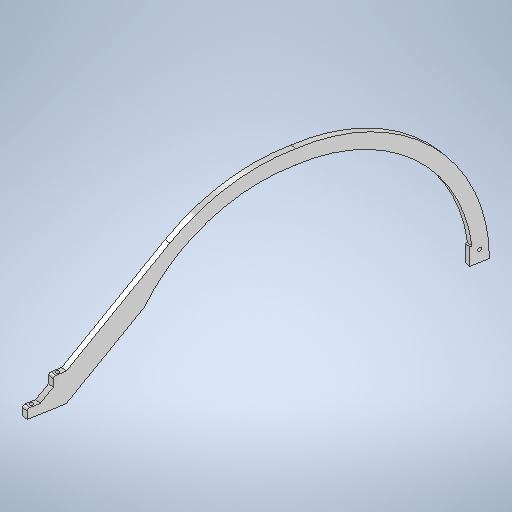
# Autodesk Inventor part: hand2_06
Saved by Autodesk Inventor 2025.1 (Build 291241000, 241)
## iProperties
Created: 2025-02-02
Part Number: hand2_06
Material: アルミニウム 6061-AHC
Document SubType Name: Modeling
Designer: ryogo
Density: 2.7 g/cm^3
Appearance: アルミニウム - ダーク
Author: ryogo
Autodesk Inventor part; units mm, degrees
ref_plane "YZ Plane" through (0, 0, 0) normal (1, 0, 0) x (0, 1, 0)
ref_plane "XZ Plane" through (0, 0, 0) normal (0, 1, 0) x (-1, 0, 0)
ref_plane "XY Plane" through (0, 0, 0) normal (0, 0, 1) x (1, 0, 0)
sketch "スケッチ1" plane through (0, 0, 0) normal (0, 1, 0) x (-1, 0, 0)
  circle A0 centre (0, 0) radius 122.5
  line L0 (0, 0) -> (21.2719, 120.6389)
  line L1 (21.2719, 120.6389) -> (-21.2719, -120.6389)
  line L2 (21.2719, 120.6389) -> (-41.166, -233.4643)
  arc A1 (21.2719, 120.6389) -> (0, 122.5) centre (0, 0) ccw
  arc A2 (-21.2719, -120.6389) -> (0, -122.5) centre (0, 0) ccw
  arc A3 (-41.8975, -115.1123) -> (-21.2719, -120.6389) centre (0, 0) ccw
  circle A4 centre (0, 0) radius 125
  circle A5 centre (0, 0) radius 145
  arc A6 (-42.7525, -117.4616) -> (-105.9051, -66.4011) centre (0, 0) ccw
  line L3 (0, 0) -> (-42.7525, -117.4616) construction
  line L4 (21.706, 123.101) -> (21.706, 123.101)
  line L5 (0, -145) -> (0, -265.735)
  line L6 (0, 0) -> (-41.8975, -115.1123)
  line L7 (-49.5929, -136.2554) -> (-41.8975, -115.1123)
  line L8 (-42.7525, -117.4616) -> (-231.4975, -48.764)
  line L9 (42.7525, 117.4616) -> (0, 0)
  line L10 (0, -145) -> (0, 145)
  line L11 (0, 0) -> (0, 300)
  circle A7 centre (0, 300) radius 20
  line L12 (117.0937, 43.75) -> (18.735, 307)
  line L13 (0, 0) -> (185.4327, 0)
  line L14 (0, 0) -> (-259.4726, 94.4403)
  line L15 (42.7525, 117.4616) -> (-253.7236, 225.3701)
  line L16 (0, 125) -> (22.0409, 125)
  line L17 (21.2719, 120.6389) -> (25.179, 142.7971)
  line L18 (42.7525, 117.4616) -> (65.8461, 180.9106)
  line L19 (15, 170) -> (69.9226, 170)
  line L20 (15.9946, 175) -> (68.0545, 175)
  line L21 (0, 125) -> (-15, 125)
  line L22 (-15, 125) -> (-15, 325)
  line L23 (-15, 325) -> (0, 325)
  line L24 (0, 325) -> (0, 125)
  line L25 (0, 125) -> (15, 125)
  line L26 (15, 125) -> (15, 325)
  line L27 (15, 325) -> (0, 325)
  line L28 (0, 325) -> (0, 125)
  line L29 (15, 200) -> (15, 325)
  line L30 (15, 325) -> (-15, 325)
  line L31 (-15, 325) -> (-15, 150)
  line L32 (15, 170) -> (37.5, 170)
  line L33 (37.5, 170) -> (17.5, 170)
  line L34 (0, 0) -> (0, 300)
  line L35 (0, -125) -> (42.7525, 117.4616)
  line L36 (-42.7525, -117.4616) -> (0, 125)
  line L37 (0, -125) -> (-3.519, -144.9573)
  line L38 (42.7525, 117.4616) -> (49.5929, 136.2554)
  line L39 (0, 125) -> (3.519, 144.9573)
  line L40 (-42.7525, -117.4616) -> (-46.2715, -137.4189)
  line L41 (42.7525, 117.4616) -> (46.2715, 137.4189)
  line L42 (-3.519, -144.9573) -> (46.2715, 137.4189)
  line L43 (46.2715, 137.4189) -> (37.2054, 139.0175)
  line L44 (-12.5852, -143.3587) -> (-3.519, -144.9573)
  line L45 (-46.2715, -137.4189) -> (3.519, 144.9573)
  line L46 (3.519, 144.9573) -> (12.5852, 143.3587)
  line L47 (-37.2054, -139.0175) -> (-46.2715, -137.4189)
  line L48 (-27.6373, -142.3418) -> (-22.7132, -143.21)
  line L49 (-27.6373, -142.3418) -> (-22.7132, -143.21)
  line L50 (-22.7132, -143.21) -> (27.641, 142.363)
  line L51 (27.641, 142.363) -> (22.717, 143.2312)
  line L52 (22.717, 143.2312) -> (-27.6373, -142.3418)
  line L53 (12.5852, 143.3587) -> (-37.2054, -139.0175)
  line L54 (-12.5852, -143.3587) -> (37.2054, 139.0175)
  line L55 (-42.1294, -138.1492) -> (7.6611, 144.2269)
  line L56 (-7.6611, -144.2269) -> (42.1294, 138.1492)
  line L57 (12.5852, 143.3587) -> (7.6611, 144.2269)
  line L58 (7.6611, 144.2269) -> (29.236, 266.5842)
  line L59 (29.236, 266.5842) -> (34.1601, 265.7159)
  line L60 (34.1601, 265.7159) -> (12.5852, 143.3587)
  line L61 (22.717, 143.2312) -> (25.179, 142.7971)
  line L62 (25.179, 142.7971) -> (42.462, 240.8141)
  line L63 (42.462, 240.8141) -> (40, 241.2482)
  line L64 (40, 241.2482) -> (22.717, 143.2312)
  line L65 (42.1294, 138.1492) -> (37.2054, 139.0175)
  line L66 (37.2054, 139.0175) -> (49.9319, 211.1932)
  line L67 (49.9319, 211.1932) -> (54.8559, 210.3249)
  line L68 (54.8559, 210.3249) -> (42.1294, 138.1492)
  line L69 (25.179, 142.7971) -> (27.641, 142.363)
  line L70 (27.641, 142.363) -> (44.508, 238.0204)
  line L71 (44.508, 238.0204) -> (42.046, 238.4546)
  line L72 (42.046, 238.4546) -> (25.179, 142.7971)
  line L73 (15.9946, 175) -> (15, 175)
  line L74 (15, 175) -> (0, 175)
  line L75 (0, 175) -> (0, 170)
  line L76 (0, 170) -> (15, 170)
  line L77 (15, 170) -> (15, 175)
  line L78 (20, 175) -> (40, 175)
  line L79 (40, 175) -> (40, 245)
  line L80 (40, 245) -> (20, 245)
  line L81 (20, 245) -> (20, 175)
  line L82 (30, 175) -> (30, 118.7697)
  line L83 (0, 175) -> (58.7137, 175)
  line L84 (58.7137, 175) -> (58.7137, 200)
  line L85 (58.7137, 200) -> (0, 200)
  line L86 (0, 200) -> (0, 175)
  line L87 (0, 200) -> (50, 200)
  line L88 (50, 200) -> (50, 170)
  line L89 (50, 170) -> (0, 170)
  line L90 (0, 170) -> (0, 200)
  line L91 (50, 170) -> (0, 170)
  line L92 (0, 170) -> (0, 165)
  line L93 (0, 200) -> (-15, 200)
  line L94 (-15, 200) -> (-15, 180)
  line L95 (-15, 180) -> (0, 180)
  line L96 (0, 180) -> (0, 200)
  line L97 (0, 180) -> (-15, 180)
  line L98 (-15, 180) -> (-15, 175)
  line L99 (-15, 175) -> (0, 175)
  line L100 (0, 175) -> (0, 180)
  line L101 (0, 145) -> (-15, 145)
  line L102 (-15, 145) -> (-20.5, 145)
  line L103 (-20.5, 145) -> (-20.5, 200)
  line L104 (-20.5, 200) -> (-15, 200)
  line L105 (-15, 200) -> (-15, 145)
  line L106 (-20.5, 150) -> (-25, 150)
  line L107 (-25, 150) -> (-25, 180)
  line L108 (-25, 180) -> (-20.5, 180)
  line L109 (-20.5, 180) -> (-20.5, 150)
  line L110 (50, 175) -> (-15, 175)
  line L111 (-15, 175) -> (-15, 170)
  line L112 (50, 170) -> (50, 175)
  line L113 (-20.5, 165) -> (-25, 165)
  line L114 (-25, 165) -> (-25, 195)
  line L115 (-25, 195) -> (-20.5, 195)
  line L116 (-20.5, 195) -> (-20.5, 165)
  line L117 (15, 250) -> (-15, 250)
  line L118 (-15, 145) -> (15, 145)
  line L119 (31.698, 266.1501) -> (-39.6674, -138.5834)
  line L120 (52.3939, 210.7591) -> (-10.1232, -143.7928)
  line L121 (49.3441, 179.0659) -> (14.8758, 185.1436)
  line L122 (-15, 138.4818) -> (-15, 121.5782)
  line L123 (-7.6611, -144.2269) -> (-42.1294, -138.1492)
  line L124 (-39.6243, -123.9424) -> (-5.1561, -130.02)
  line L125 (-42.2291, -138.7145) -> (-7.7608, -144.7922)
  line L126 (-41.3608, -133.7904) -> (-6.8926, -139.8681)
  line L127 (-6.0243, -134.9441) -> (-40.4926, -128.8664)
  line L128 (18.3488, 204.8397) -> (52.8171, 198.762)
  line L129 (50.2124, 183.9899) -> (45.0029, 154.4457)
  line L130 (10.5346, 160.5234) -> (15.7441, 190.0676)
  line L131 (19.217, 209.7638) -> (53.6853, 203.6861)
  line L132 (15, 250) -> (53.6853, 203.6861)
  line L133 (53.6853, 203.6861) -> (53.6853, 170)
  line L134 (53.6853, 170) -> (-15, 170)
  line L135 (-15, 172.5) -> (53.6853, 172.5)
  line L136 (15, 170) -> (15, 150)
  line L137 (15, 150) -> (-15, 150)
  line L138 (-15, 170) -> (15, 170)
  line L139 (15, 150) -> (-15, 150)
  line L140 (-15, 150) -> (-15, 325)
  line L141 (-15, 325) -> (15, 325)
  line L142 (15, 325) -> (15, 150)
  circle A8 centre (0, 300) radius 6
  circle A9 centre (0, 300) radius 11
  line L143 (47.7456, 170) -> (15, 150)
  point P0 (-25.1752, -142.7759)
  point P1 (42.3116, 114.9608)
  point P2 (0, 133.0222)
  point P3 (-38.8988, -134.2246)
  point P4 (-38.0306, -129.3005)
  point P5 (-23.2585, -131.9052)
  point P6 (-24.1267, -136.8293)
  point P7 (-9.3546, -139.434)
  point P8 (-8.4863, -134.51)
  point P9 (17.3379, 184.7094)
  point P10 (32.11, 182.1047)
  point P11 (46.8821, 179.5)
  point P12 (50.3551, 199.1962)
  point P13 (35.5829, 201.8009)
  point P14 (20.8108, 204.4056)
  point P15 (0, 240)
  point P16 (0, 190)
  point P17 (0, 289)
  point P18 (0, 311)
  point P19 (37.5, 172.5)
  point P20 (22.5, 172.5)
  point P21 (-22.4332, -141.6222)
  point P22 (-19.9282, -127.4153)
  point P23 (-24.8522, -126.5471)
  point P24 (-27.3573, -140.754)
  dimension "d0" = 245
  dimension "d7" = 290
  dimension "d19" = 40
  dimension "d1" = 0
  dimension "d4" = 42.5438
  dimension "d5" = 21.3532
  dimension "d6" = 250
  dimension "d10" = 0
  dimension "d12" = 0
  dimension "d13" = 10
  dimension "d15" = 0
  dimension "d16" = 9.8877
  dimension "d18" = 10
  dimension "d21" = 145
  dimension "d23" = 175
  dimension "d26" = 7.5384
  dimension "d30" = 180
  dimension "d34" = 180
  dimension "d35" = 45
  dimension "d37" = 5
  dimension "d38" = 15
  dimension "d39" = 200
  dimension "d40" = 15
  dimension "d41" = 200
  dimension "d47" = 300
  dimension "d52" = 5
  dimension "d53" = 0
  dimension "d54" = 10
  dimension "d55" = 10
  dimension "d56" = 5
  dimension "d57" = 5
  dimension "d60" = 5
  dimension "d61" = 20
  dimension "d62" = 70
  dimension "d63" = 5
  dimension "d65" = 25
  dimension "d66" = 50
  dimension "d68" = 20
  dimension "d69" = 5
  dimension "d74" = 20
  dimension "d75" = 5.5
  dimension "d76" = 55
  dimension "d77" = 4.5
  dimension "d78" = 30
  dimension "d79" = 5
  dimension "d82" = 15
  dimension "d83" = 50
  dimension "d87" = 16.9036
  dimension "d88" = 10.0392
  dimension "d89" = 10.5222
  dimension "d92" = 15
  dimension "d93" = 5
  dimension "d94" = 5
  dimension "d96" = 4.5
  dimension "d97" = 5
  dimension "d98" = 30
  dimension "d99" = 10
  dimension "d101" = 20
  dimension "d102" = 10
  dimension "d103" = 20
  dimension "d104" = 12
  dimension "d105" = 22
  dimension "d106" = 7.5
  dimension "d107" = 15
  dimension "d108" = 30
  constraints: 287 end point, 87 point on line, 44 parallel, 39 perpendicular, 19 horizontal, 16 point on circle, 14 midpoint, 9 coincident, 9 collinear, 7 centre point, 3 vertical, 2 tangent, 1 symmetric about line, 43 other
  measures "d1" horizontal distance of point (0, 0) A2.end
  measures "d4" distance of L6.end A2.end
  measures "d5" distance of A1.end L0.end
  measures "d6" diameter of A4
  measures "d10" horizontal distance of A4.centre L16.start
  measures "d12" distance from line of L5 point (0, 0)
  measures "d15" horizontal distance of A2.end L35.start
  measures "d16" vertical distance of L6.end L35.start
  measures "d18" angle of L9 L1
  measures "d21" distance of L5.start A2.centre
  measures "d23" distance of L11.end L16.start
  measures "d26" distance from line of L15 L16.start
  measures "d30" angle of L4 L17
  measures "d34" angle of L9 L18
  measures "d35" distance from line of L19 L16.start
  measures "d37" distance between parallel lines of L19 L20
  measures "d38" distance of L22.end L23.end
  measures "d39" distance of L21.end L22.end
  measures "d40" distance of L27.end L26.end
  measures "d41" distance from line of L16.start L27
  measures "d47" distance of L3.start L11.end
  measures "d52" distance of L48.start L48.end
  measures "d53" distance from line of L2 point (-25.175, -142.776)
  measures "d54" distance between parallel lines of L52 L53
  measures "d55" distance between parallel lines of L54 L50
  measures "d56" distance of L46.end L55.end
  measures "d57" distance of L43.end L56.end
  measures "d60" distance between parallel lines of L76 L74
  measures "d61" distance of L80.end L79.end
  measures "d62" distance of L79.end L78.end
  measures "d63" distance between parallel lines of L26 L81
  measures "d65" distance of L84.end L83.end
  measures "d66" distance of L88.end L89.end
  measures "d68" distance between parallel lines of L95 L93
  measures "d69" distance between parallel lines of L99 L97
  measures "d74" distance of L16.start L101.start
  measures "d75" distance of L103.end L104.end
  measures "d76" distance of L102.end L103.end
  measures "d77" distance of L107.end L108.end
  measures "d78" distance of L106.end L107.end
  measures "d79" distance between parallel lines of L102 L106
  measures "d82" distance between parallel lines of L106 L113
  measures "d83" distance between parallel lines of L93 L117
  measures "d87" distance of L122.start L122.end
  measures "d88" vertical distance of point (42.312, 114.961) L25.end
  measures "d89" distance of A1.end point (0, 133.022)
  measures "d92" distance of L125.start L124.start
  measures "d93" distance of L125.start L126.start
  measures "d94" distance of L127.end L124.start
  measures "d96" distance from line of L20 point (46.882, 179.5)
  measures "d97" distance of L121.end L130.end
  measures "d98" distance of L129.start L129.end
  measures "d99" distance from line of L117 point (0, 240)
  measures "d101" distance of L128.start L121.end
  measures "d102" diameter of L131 L128
  measures "d103" distance of L19.start L136.end
  measures "d104" diameter of A8
  measures "d105" diameter of A9
  measures "d106" distance from line of point (22.5, 172.5) L142
  measures "d107" distance of point (22.5, 172.5) point (37.5, 172.5)
  measures "d108" distance between parallel lines of L113 L115
extrude "押し出し1" add sketch "スケッチ1" along normal blind 5 contours L123 L2 L126 L50 | L50 L127 L2 L124 | L126 L2 L127 L50 | L123 L52 L126 L2 | L2 L127 L52 L124 | L126 L52 L127 L2
sketch "スケッチ3" plane through (19.9282, 0, -127.4153) normal (-0.9848078, 0, -0.1736482) x (-0.1736482, 0, 0.9848078)
  line L0 (253.9401, 0) -> (3.9401, 0) projected
  circle A0 centre (128.9401, 0) radius 132.5
  circle A1 centre (128.9401, 0) radius 145
  circle A2 centre (136.4401, 0) radius 132.5
  circle A3 centre (136.4401, 0) radius 145
  line L1 (128.9401, -145) -> (136.4401, -145)
  line L2 (128.9401, -132.5) -> (136.4401, -132.5)
  line L3 (-16.0599, 0) -> (281.4401, 0)
  line L4 (-14.426, 0) -> (0, 0) projected
  point P0 (128.9401, 0)
  point P1 (132.6901, 144.9515)
  point P2 (-3.5599, 0)
  point P3 (132.6901, 132.4469)
  point P4 (268.9401, 0)
  point P5 (3.9401, 0)
  dimension "d112" = 265
  dimension "d114" = 265
  dimension "d113" = 290
  dimension "d115" = 290
  dimension "d116" = 7.5
  dimension "d117" = 0
  constraints: 6 end point, 4 point on circle, 3 coincident, 3 horizontal, 2 centre point, 1 collinear, 1 point on line, 1 tangent, 6 other
  measures "d113" diameter of A1
  measures "d115" diameter of A3
  measures "d116" distance of point (128.94, 0) point (136.44, 0)
  measures "d117" distance from line of L0 L3.end
extrude "押し出し2" add sketch "スケッチ3" against normal blind 5 contours A0 L3 A3 A1 A2 | A1 A3 L3 | L3 A1 A3 picked at (278.6261, 5.5003) picked at (-11.7, 21.7524)
sketch "スケッチ4" plane through (-3.7644, 0, 6.9519) normal (-0.9848078, 0, -0.1736482) x (-0.1243654, -0.6979033, 0.7053115)
  line L0 (98.4764, 95.9617) -> (168.0424, 163.7512) projected
  line L1 (127.0625, 123.8178) -> (123.4815, 120.3283)
  line L2 (123.4815, 120.3283) -> (109.5235, 134.6521)
  line L3 (109.5235, 134.6521) -> (113.1044, 138.1416)
  line L4 (113.1044, 138.1416) -> (127.0625, 123.8178)
  line L5 (141.3863, 137.7759) -> (144.9673, 141.2654)
  line L6 (144.9673, 141.2654) -> (131.0092, 155.5892)
  line L7 (131.0092, 155.5892) -> (127.4283, 152.0997)
  line L8 (127.4283, 152.0997) -> (141.3863, 137.7759)
  line L9 (113.1044, 138.1416) -> (127.0625, 123.8178)
  line L10 (127.0625, 123.8178) -> (141.3863, 137.7759)
  line L11 (141.3863, 137.7759) -> (127.4283, 152.0997)
  line L12 (127.4283, 152.0997) -> (113.1044, 138.1416)
  line L13 (131.0092, 155.5892) -> (-11.2051, 144.5664)
  arc A0 (103.8478, 101.196) -> (-103.8478, 101.196) centre (0, 0) ccw projected
  line L14 (109.5235, 134.6521) -> (62.1952, 130.9838)
  line L15 (62.1952, 130.9838) -> (31.7985, 128.6278)
  arc A1 (94.8954, 92.4722) -> (-95.1209, 92.2403) centre (0, 0) ccw projected
  line L16 (131.0092, 155.5892) -> (127.4283, 152.0997)
  line L17 (113.1044, 138.1416) -> (109.5235, 134.6521)
  line L18 (109.5235, 134.6521) -> (92.0626, 152.5705)
  line L19 (92.0626, 152.5705) -> (95.6436, 156.06)
  line L20 (95.6436, 156.06) -> (113.1044, 138.1416)
  line L21 (113.1044, 138.1416) -> (95.6436, 156.06)
  line L22 (95.6436, 156.06) -> (99.2245, 159.5496)
  line L23 (99.2245, 159.5496) -> (116.6854, 141.6312)
  line L24 (116.6854, 141.6312) -> (113.1044, 138.1416)
  line L25 (127.4283, 152.0997) -> (123.8473, 148.6102)
  line L26 (123.8473, 148.6102) -> (118.027, 154.583)
  line L27 (118.027, 154.583) -> (121.608, 158.0725)
  line L28 (121.608, 158.0725) -> (127.4283, 152.0997)
  line L29 (131.0092, 155.5892) -> (127.4283, 152.0997)
  line L30 (127.4283, 152.0997) -> (121.608, 158.0725)
  line L31 (121.608, 158.0725) -> (125.1889, 161.562)
  line L32 (125.1889, 161.562) -> (131.0092, 155.5892)
  point P0 (-5.3714, -5.2343)
  point P1 (127.0625, 123.8178)
  point P2 (141.3863, 137.7759)
  point P3 (144.9673, 141.2654)
  point P4 (127.4283, 152.0997)
  point P5 (131.0092, 155.5892)
  point P6 (105.0448, 153.5768)
  dimension "d120" = 20
  dimension "d121" = 5
  dimension "d122" = 20
  dimension "d123" = 180
  dimension "d124" = 5
  dimension "d125" = 5
  dimension "d126" = 0
  dimension "d127" = 8.3397
  constraints: 64 end point, 15 parallel, 7 perpendicular, 5 collinear, 3 point on circle, 3 point on line, 1 tangent, 3 other
  measures "d120" distance of L1.end L2.end
  measures "d121" distance between parallel lines of L4 L2
  measures "d122" distance of the line from the sketch origin of L7
  measures "d123" angle of L14 L15
  measures "d124" distance of L19.end L22.end
  measures "d125" distance of L11.end L25.end
  measures "d126" distance between parallel lines of L6 L32
  measures "d127" distance between parallel lines of L12 L27
extrude "押し出し3" add sketch "スケッチ4" against normal blind 5 contours A0 L13 L18 L14 | L18 L13 L20 L3 | L20 L13 L23 L12 | L19 L20 L13 | L28 L13 L7 | L12 L26 L13 L28 | L23 L13 L26 L12 | L20 L22 L23 L13 | L13 L28 L31 L32 | L13 L27 L28
sketch "スケッチ5" plane through (-2.462, 0, -0.4341) normal (-0.9848078, 0, -0.1736482) x (-0.1243654, 0.6979033, 0.7053115)
  line L0 (137.9199, -64.0212) -> (134.7786, -33.6956)
  arc A0 (100.2669, -97.7065) -> (95.1209, 92.2403) centre (5.3714, -5.2343) ccw projected
  line L1 (137.9199, -64.0212) -> (142.811, -111.2387) projected
  line L2 (-103.8478, 101.196) -> (-92.3459, 89.9877) projected
  line L3 (-92.3459, 89.9877) -> (-88.8564, 93.5687) projected
  line L4 (-91.3383, 95.9873) -> (-88.8564, 93.5687) projected
  arc A1 (95.1209, 92.2403) -> (-91.3383, 95.9873) centre (0, 0) ccw projected
  arc A2 (100.2669, -97.7065) -> (95.1209, 92.2403) centre (5.3714, -5.2343) ccw projected
  line L5 (100.2669, -97.7065) -> (109.2193, -106.4302) projected
  arc A3 (109.2193, -106.4302) -> (137.9199, -64.0212) centre (5.3714, -5.2343) ccw projected
  line L6 (137.9199, -64.0212) -> (142.811, -111.2387) projected
  line L7 (142.811, -111.2387) -> (164.2968, -132.1758) projected
  line L8 (164.2968, -132.1758) -> (170.1171, -126.203) projected
  line L9 (170.1171, -126.203) -> (162.9551, -119.224) projected
  line L10 (162.9551, -119.224) -> (161.6135, -106.2721) projected
  line L11 (161.6135, -106.2721) -> (167.4338, -100.2993) projected
  line L12 (167.4338, -100.2993) -> (160.2719, -93.3203) projected
  line L13 (160.2719, -93.3203) -> (149.5997, 9.7059) projected
  arc A4 (149.5997, 9.7059) -> (103.8478, 101.196) centre (5.3714, -5.2343) ccw projected
  arc A5 (103.8478, 101.196) -> (-103.8478, 101.196) centre (0, 0) ccw projected
  point P0 (0, 0)
  point P1 (100.2669, -97.7065)
  constraints: 2 end point, 1 collinear, 1 point on circle
extrude "押し出し4" cut sketch "スケッチ5" against normal blind 5 contours A3 L5 A0 L0
sketch "スケッチ6" plane through (-2.462, 0, -0.4341) normal (-0.9848078, 0, -0.1736482) x (-0.1243654, 0.6979033, 0.7053115)
  line L0 (134.7786, -33.6956) -> (142.811, -111.2387) projected
  line L1 (142.811, -111.2387) -> (164.2968, -132.1758) projected
  line L2 (164.2968, -132.1758) -> (170.1171, -126.203) projected
  line L3 (170.1171, -126.203) -> (162.9551, -119.224) projected
  line L4 (162.9551, -119.224) -> (161.6135, -106.2721) projected
  line L5 (161.6135, -106.2721) -> (167.4338, -100.2993) projected
  line L6 (167.4338, -100.2993) -> (160.2719, -93.3203) projected
  line L7 (160.2719, -93.3203) -> (149.5997, 9.7059) projected
  arc A0 (149.5997, 9.7059) -> (103.8478, 101.196) centre (5.3714, -5.2343) ccw projected
  arc A1 (103.8478, 101.196) -> (-103.8478, 101.196) centre (0, 0) ccw projected
  line L8 (-103.8478, 101.196) -> (-92.3459, 89.9877) projected
  line L9 (-92.3459, 89.9877) -> (-88.8564, 93.5687) projected
  line L10 (-91.3383, 95.9873) -> (-88.8564, 93.5687) projected
  arc A2 (95.1209, 92.2403) -> (-91.3383, 95.9873) centre (0, 0) ccw projected
  arc A3 (134.7786, -33.6956) -> (95.1209, 92.2403) centre (5.3714, -5.2343) ccw projected
  circle A4 centre (0, 0) radius 132.5 projected
  point P0 (0, 0)
extrude "押し出し5" cut sketch "スケッチ3" against normal blind 5 contours L3 A0 A2 picked at (4.1359, 25.6132)
sketch "スケッチ7" plane through (-2.462, 0, -0.4341) normal (-0.9848078, 0, -0.1736482) x (-0.1243654, 0.6979033, 0.7053115)
  line L0 (-94.8954, 92.4722) -> (-103.8478, 101.196) projected
  line L1 (-103.8478, 101.196) -> (-93.3793, 111.9389)
  line L2 (-93.3793, 111.9389) -> (-82.6364, 101.4703)
  line L3 (-82.6364, 101.4703) -> (-93.105, 90.7274)
  line L4 (-93.105, 90.7274) -> (-103.8478, 101.196)
  arc A0 (103.8478, 101.196) -> (-103.8478, 101.196) centre (0, 0) ccw projected
  point P0 (0, 0)
  point P1 (-92.8221, 111.3959)
  point P2 (-94.8954, 92.4722)
  dimension "d134" = 15
  dimension "d135" = 15
  constraints: 8 end point, 2 parallel, 1 perpendicular, 1 tangent
  measures "d134" distance of L0.end L1.end
  measures "d135" distance between parallel lines of L3 L1
extrude "押し出し6" add sketch "スケッチ7" against normal blind 5 contours L0 A0 L2 L3 L4
sketch "スケッチ8" plane through (-35.4402, 45.019, 186.5946) normal (0, 1, 0) x (0.9848078, 0, 0.1736482)
  line L0 (0, 0) -> (0, 10) projected
  line L1 (0, 0) -> (5, 0) projected
  line L2 (5, 10) -> (5, 0) projected
  line L3 (0, 10) -> (5, 10) projected
  line L4 (0, -20) -> (0, -10) projected
  line L5 (0, -20) -> (5, -20) projected
  line L6 (5, -10) -> (5, -20) projected
  line L7 (0, -10) -> (5, -10) projected
  point P0 (2.5, 189.914)
  point P1 (2.5, 5)
  point P2 (2.5, -15)
  dimension "d138" = 2.5
  dimension "d139" = 5
  dimension "d140" = 2.5
  dimension "d141" = 5
  measures "d138" distance from line of L2 point (2.5, 5)
  measures "d139" vertical distance of L1.end point (2.5, 5)
  measures "d140" distance from line of L6 point (2.5, -15)
  measures "d141" distance from line of L5 point (2.5, -15)
hole "穴1" at (-32.11, 45.019, 182.1047) at (-35.5829, 45.019, 201.8009) direction (0, -1, 0) diameter 3.1 end through all
fillet "フィレット1" radius 2 2 edges at (-32.9782, 45.019, 187.0288) (-36.4512, 28.3397, 206.7249)
sketch "スケッチ9" plane through (25.0363, 0, -127.5909) normal (0.9848078, 0, 0.1736482) x (0.1736482, 0, -0.9848078)
  line L0 (0, 15) -> (0, 0) projected
  line L1 (0, 0) -> (15, 0) projected
  point P0 (-130, 0)
  point P1 (7.5, 10)
  dimension "d150" = 7.5
  dimension "d151" = 10
  measures "d150" distance from line of L0 point (7.5, 10)
  measures "d151" distance from line of L1 point (7.5, 10)
hole "穴2" at (26.3386, 10, -134.9769) direction (-0.9848078, 0, -0.1736482) diameter 3.1 end through all
equation "\"d18\" = d13"
